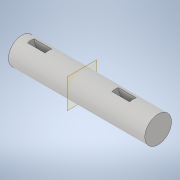
# Autodesk Inventor part: MotorShaft
Saved by Autodesk Inventor 2021 (Build 250183000, 183)
## iProperties
Created: 2020-09-20
Part Number: MotorShaft
Material: Generic
Document SubType Name: Modeling
Designer: PhotonUser
Density: 1 g/cm^3
Appearance: Default
Author: PhotonUser
Autodesk Inventor part; units mm, degrees
ref_plane "YZ Plane" through (0, 0, 0) normal (1, 0, 0) x (0, 1, 0)
ref_plane "XZ Plane" through (0, 0, 0) normal (0, 1, 0) x (-1, 0, 0)
ref_plane "XY Plane" through (0, 0, 0) normal (0, 0, 1) x (1, 0, 0)
sketch "Sketch1" plane through (0, 0, 0) normal (1, 0, 0) x (0, 1, 0)
  circle A0 centre (0, 0) radius 9.525
  dimension "d0" = 19.05
  constraints: 1 centre point, 1 coincident
  measures "d0" diameter of A0
extrude "Extrusion1" add sketch "Sketch1" along normal blind 85.725
sketch "Sketch3" plane through (0, 0, 0) normal (0, 0, 1) x (1, 0, 0)
  line L0 (0, 9.525) -> (85.725, 9.525) projected
  arc A0 (6.35, 9.525) -> (19.05, 9.525) centre (12.7, 9.525) ccw
  line L1 (6.35, 9.525) -> (19.05, 9.525)
  point P0 (0, 0)
  dimension "d7" = 12.7
  dimension "d8" = 12.7
  constraints: 3 point on line, 2 end point, 2 point on circle, 1 centre point
  measures "d7" distance of L0.start A0.centre
  measures "d8" diameter of A0
extrude "Extrusion3" cut sketch "Sketch3" against normal mid plane 4.7752
ref_plane "Work Plane1" through (42.8561, 0, 0) normal (1, 0, 0) x (0, 0, -1)
mirror "Mirror1" about plane through (42.8561, 0, 0) normal (1, 0, 0) of "Extrusion3"
sketch "Sketch4" plane through (85.725, 0, 0) normal (1, 0, 0) x (0, 0, -1)
  circle A0 centre (0, 0) radius 9.525
  constraints: 1 centre point, 1 coincident
extrude "Extrusion4" add sketch "Sketch4" along normal blind 11.6586
body "Solid1"
